generated POWER BOX WITH BOX OPERATIONS 7uncut_v3 (Autodesk Fusion 360 design; units mm, degrees)
Autodesk Fusion 360 part; units mm, degrees
(part 1 of 2)
sketch "b  stock" plane through (0, 0, 0) normal (0, 0, 1) x (1, 0, 0)
  line L0 (0, 0) -> (304.8, 0)
  line L1 (304.8, 0) -> (304.8, 609.6)
  line L2 (304.8, 609.6) -> (0, 609.6)
  line L3 (0, 609.6) -> (0, 0)
extrude "b  stock body extrude Feature" add sketch "b  stock" along normal blind 3.175 makes body 1
sketch "b  layout" plane through (0, 0, 0) normal (0, 0, 1) x (1, 0, 0)
  line L0 (0, 0) -> (90, 0)
  line L1 (90, 0) -> (90, 85)
  line L2 (90, 85) -> (0, 85)
  line L3 (0, 85) -> (0, 0)
  line L4 (92.01, 0) -> (182.01, 0)
  line L5 (182.01, 0) -> (182.01, 85)
  line L6 (182.01, 85) -> (92.01, 85)
  line L7 (92.01, 85) -> (92.01, 0)
  line L8 (184.02, 0) -> (234.02, 0)
  line L9 (234.02, 0) -> (234.02, 85)
  line L10 (234.02, 85) -> (184.02, 85)
  line L11 (184.02, 85) -> (184.02, 0)
  line L12 (236.03, 0) -> (286.03, 0)
  line L13 (286.03, 0) -> (286.03, 85)
  line L14 (286.03, 85) -> (236.03, 85)
  line L15 (236.03, 85) -> (236.03, 0)
  line L16 (0, 87.01) -> (90, 87.01)
  line L17 (90, 87.01) -> (90, 137.01)
  line L18 (90, 137.01) -> (0, 137.01)
  line L19 (0, 137.01) -> (0, 87.01)
  line L20 (92.01, 87.01) -> (182.01, 87.01)
  line L21 (182.01, 87.01) -> (182.01, 137.01)
  line L22 (182.01, 137.01) -> (92.01, 137.01)
  line L23 (92.01, 137.01) -> (92.01, 87.01)
sketch "top content" plane through (0, 0, 0) normal (0, 0, 1) x (1, 0, 0) in component "b top component"
  line L0 (0, 85) -> (90, 85) construction
  line L1 (90, 0) -> (0, 0) construction
  line L2 (14.1663, 44.1604) -> (78.1663, 44.1604) construction
  line L3 (78.1663, 44.1604) -> (78.1663, 63.1604) construction
  line L4 (78.1663, 63.1604) -> (14.1663, 63.1604) construction
  line L5 (14.1663, 63.1604) -> (14.1663, 44.1604) construction
  line L6 (0, 0) -> (0, 85) construction
  dimension "d1818" = 15
  dimension "d1163" = 90
  dimension "d1817" = 85
  constraint horizontal L0
  constraint perpendicular L1 L6
  measures "d1163" distance of L0.start L0.end
  measures "d1817" distance of L1.start L0.end
sketch "b top lines" plane through (0, 0, 0) normal (0, 0, 1) x (1, 0, 0) in component "b top component"
  line L0 (0, 0) -> (10.1, 0)
  line L1 (10.1, 0) -> (10.1, 3.175)
  line L2 (10.1, 3.175) -> (19.9, 3.175)
  line L3 (19.9, 3.175) -> (19.9, 0)
  line L4 (19.9, 0) -> (30.1, 0)
  line L5 (30.1, 0) -> (30.1, 3.175)
  line L6 (30.1, 3.175) -> (39.9, 3.175)
  line L7 (39.9, 3.175) -> (39.9, 0)
  line L8 (39.9, 0) -> (50.1, 0)
  line L9 (50.1, 0) -> (50.1, 3.175)
  line L10 (50.1, 3.175) -> (59.9, 3.175)
  line L11 (59.9, 3.175) -> (59.9, 0)
  line L12 (59.9, 0) -> (70.1, 0)
  line L13 (70.1, 0) -> (70.1, 3.175)
  line L14 (70.1, 3.175) -> (79.9, 3.175)
  line L15 (79.9, 3.175) -> (79.9, 0)
  line L16 (79.9, 0) -> (90, 0)
  line L17 (90, 0) -> (90, 17.6)
  line L18 (90, 17.6) -> (86.825, 17.6)
  line L19 (86.825, 17.6) -> (86.825, 27.4)
  line L20 (86.825, 27.4) -> (90, 27.4)
  line L21 (90, 27.4) -> (90, 37.6)
  line L22 (90, 37.6) -> (86.825, 37.6)
  line L23 (86.825, 37.6) -> (86.825, 47.4)
  line L24 (86.825, 47.4) -> (90, 47.4)
  line L25 (90, 47.4) -> (90, 57.6)
  line L26 (90, 57.6) -> (86.825, 57.6)
  line L27 (86.825, 57.6) -> (86.825, 67.4)
  line L28 (86.825, 67.4) -> (90, 67.4)
  line L29 (90, 67.4) -> (90, 85)
  line L30 (0, 85) -> (10.1, 85)
  line L31 (10.1, 85) -> (10.1, 81.825)
  line L32 (10.1, 81.825) -> (19.9, 81.825)
  line L33 (19.9, 81.825) -> (19.9, 85)
  line L34 (19.9, 85) -> (30.1, 85)
  line L35 (30.1, 85) -> (30.1, 81.825)
  line L36 (30.1, 81.825) -> (39.9, 81.825)
  line L37 (39.9, 81.825) -> (39.9, 85)
  line L38 (39.9, 85) -> (50.1, 85)
  line L39 (50.1, 85) -> (50.1, 81.825)
  line L40 (50.1, 81.825) -> (59.9, 81.825)
  line L41 (59.9, 81.825) -> (59.9, 85)
  line L42 (59.9, 85) -> (70.1, 85)
  line L43 (70.1, 85) -> (70.1, 81.825)
  line L44 (70.1, 81.825) -> (79.9, 81.825)
  line L45 (79.9, 81.825) -> (79.9, 85)
  line L46 (79.9, 85) -> (90, 85)
  line L47 (0, 0) -> (0, 17.6)
  line L48 (0, 17.6) -> (3.175, 17.6)
  line L49 (3.175, 17.6) -> (3.175, 27.4)
  line L50 (3.175, 27.4) -> (0, 27.4)
  line L51 (0, 27.4) -> (0, 37.6)
  line L52 (0, 37.6) -> (3.175, 37.6)
  line L53 (3.175, 37.6) -> (3.175, 47.4)
  line L54 (3.175, 47.4) -> (0, 47.4)
  line L55 (0, 47.4) -> (0, 57.6)
  line L56 (0, 57.6) -> (3.175, 57.6)
  line L57 (3.175, 57.6) -> (3.175, 67.4)
  line L58 (3.175, 67.4) -> (0, 67.4)
  line L59 (0, 67.4) -> (0, 85)
sketch "b top circles" plane through (0, 0, 0) normal (0, 0, 1) x (1, 0, 0) in component "b top component"
  circle A0 centre (10.6906, 2.4644) radius 1.005
  circle A1 centre (19.3094, 2.4644) radius 1.005
  circle A2 centre (30.6906, 2.4644) radius 1.005
  circle A3 centre (39.3094, 2.4644) radius 1.005
  circle A4 centre (50.6906, 2.4644) radius 1.005
  circle A5 centre (59.3094, 2.4644) radius 1.005
  circle A6 centre (70.6906, 2.4644) radius 1.005
  circle A7 centre (79.3094, 2.4644) radius 1.005
  circle A8 centre (87.5356, 18.1906) radius 1.005
  circle A9 centre (87.5356, 26.8094) radius 1.005
  circle A10 centre (87.5356, 38.1906) radius 1.005
  circle A11 centre (87.5356, 46.8094) radius 1.005
  circle A12 centre (87.5356, 58.1906) radius 1.005
  circle A13 centre (87.5356, 66.8094) radius 1.005
  circle A14 centre (10.6906, 82.5356) radius 1.005
  circle A15 centre (19.3094, 82.5356) radius 1.005
  circle A16 centre (30.6906, 82.5356) radius 1.005
  circle A17 centre (39.3094, 82.5356) radius 1.005
  circle A18 centre (50.6906, 82.5356) radius 1.005
  circle A19 centre (59.3094, 82.5356) radius 1.005
  circle A20 centre (70.6906, 82.5356) radius 1.005
  circle A21 centre (79.3094, 82.5356) radius 1.005
  circle A22 centre (2.4644, 18.1906) radius 1.005
  circle A23 centre (2.4644, 26.8094) radius 1.005
  circle A24 centre (2.4644, 38.1906) radius 1.005
  circle A25 centre (2.4644, 46.8094) radius 1.005
  circle A26 centre (2.4644, 58.1906) radius 1.005
  circle A27 centre (2.4644, 66.8094) radius 1.005
extrude "b top lines lines extrude Feature" add sketch "b top lines" along normal blind 3.175 separate body makes body 2 in component "b top component"
extrude "b top circles circles extrude Feature" add sketch "b top circles" along normal blind 3.175 separate body makes body 3 at (3.4644, 58.0906, 2.1167) makes body 4 at (3.4644, 38.0906, 2.1167) makes body 5 at (3.4644, 18.0906, 2.1167) makes body 6 at (69.7463, 82.8794, 2.1167) makes body 7 at (49.7463, 82.8794, 2.1167) makes body 8 at (31.6167, 82.926, 2.1167) makes body 9 at (9.7463, 82.8794, 2.1167) makes body 10 at (86.5913, 67.1531, 2.1167) makes body 11 at (87.2156, 45.8567, 1.0583) makes body 12 at (87.2156, 25.8567, 1.0583) makes body 13 at (78.9893, 1.5117, 1.0583) makes body 14 at (59.2843, 3.469, 2.1167) makes body 15 at (39.2843, 3.469, 2.1167) makes body 16 at (20.3094, 2.3643, 2.1167) makes body 17 at (31.6906, 2.3643, 2.1167) makes body 18 at (50.6656, 3.469, 2.1167) makes body 19 at (70.3706, 1.5117, 1.0583) makes body 20 at (87.2156, 17.238, 1.0583) makes body 21 at (87.2156, 37.238, 1.0583) makes body 22 at (87.2156, 57.238, 1.0583) makes body 23 at (11.6906, 2.3643, 2.1167) makes body 24 at (20.2354, 82.926, 2.1167) makes body 25 at (38.365, 82.8794, 2.1167) makes body 26 at (58.365, 82.8794, 2.1167) makes body 27 at (78.365, 82.8794, 2.1167) makes body 28 at (3.4644, 26.7093, 2.1167) makes body 29 at (3.4644, 46.7093, 2.1167) makes body 30 at (3.3904, 67.1997, 2.1167) in component "b top component"
combine "b top lines final combine feature" operation cut target body 2 tool bodies 3 4 5 6 7 8 9 10 11 12 13 14 15 16 17 18 19 20 21 22 23 24 25 26 27 28 29 30 in component "b top component"
sketch "bottom content" plane through (0, 0, 0) normal (0, 0, 1) x (1, 0, 0) in component "b bottom component"
  line L0 (92.01, 0) -> (182.01, 0) construction
  line L1 (182.01, 0) -> (182.01, 85) construction
  line L2 (182.01, 85) -> (92.01, 85) construction
  line L3 (92.01, 85) -> (92.01, 0) construction
  line L4 (182.01, 85) -> (182.01, 0) construction
  line L5 (182.01, 0) -> (92.01, 0) construction
  line L6 (92.01, 85) -> (182.01, 85) construction
  line L7 (92.01, 0) -> (92.01, 85) construction
  circle A0 centre (108.01, 55.5) radius 1.005
  circle A1 centre (172.01, 75) radius 1.005
  circle A2 centre (166.01, 55.5) radius 1.005
  circle A3 centre (166.01, 29.5) radius 1.005
  circle A4 centre (172.01, 10) radius 1.005
  circle A5 centre (102.01, 10) radius 1.005
  circle A6 centre (108.01, 29.5) radius 1.005
  circle A7 centre (102.01, 75) radius 1.005
  circle A8 centre (172.01, 75) radius 1.005
  point P0 (102.01, 75)
  point P1 (108.01, 55.5)
  point P2 (172.01, 75)
  point P3 (166.01, 29.5)
  point P4 (166.01, 55.5)
  point P5 (172.01, 10)
  point P6 (102.01, 10)
  point P7 (108.01, 29.5)
  point P8 (182.01, 85)
  dimension "d467" = 90
  dimension "d468" = 85
  dimension "d469" = 10
  dimension "d470" = 10
  dimension "d471" = 29.5
  dimension "d472" = 16
  dimension "d473" = 2.01
  dimension "d474" = 2.01
  constraint horizontal L5
  constraint perpendicular L5 L7
  constraint parallel L5 L6
  constraint coincident L1.end L2.start
  constraint vertical L4
  constraint coincident P1 A0.centre
  constraint coincident P2 A1.centre
  constraint coincident P4 A2.centre
  constraint coincident P3 A3.centre
  constraint coincident P5 A4.centre
  constraint coincident P6 A5.centre
  constraint coincident P7 A6.centre
  constraint coincident P0 A7.centre
  constraint concentric A1 A8
  constraint equal A0 A2
  constraint equal A7 A8
  constraint equal A0 A6
  constraint equal A0 A3
  constraint equal A3 A5
  constraint equal A3 A8
  constraint equal A2 A4
  measures "d467" distance of L1.end L2.end
  measures "d468" distance of L0.start L2.end
  measures "d469" distance of P0 L6
  measures "d470" distance of P0 L7
  measures "d471" distance of P1 L6
  measures "d472" distance of P7 L7
  measures "d473" diameter of A0
  measures "d474" diameter of A1
sketch "b bottom lines" plane through (0, 0, 0) normal (0, 0, 1) x (1, 0, 0) in component "b bottom component"
  line L0 (92.01, 0) -> (102.11, 0)
  line L1 (102.11, 0) -> (102.11, 3.175)
  line L2 (102.11, 3.175) -> (111.91, 3.175)
  line L3 (111.91, 3.175) -> (111.91, 0)
  line L4 (111.91, 0) -> (122.11, 0)
  line L5 (122.11, 0) -> (122.11, 3.175)
  line L6 (122.11, 3.175) -> (131.91, 3.175)
  line L7 (131.91, 3.175) -> (131.91, 0)
  line L8 (131.91, 0) -> (142.11, 0)
  line L9 (142.11, 0) -> (142.11, 3.175)
  line L10 (142.11, 3.175) -> (151.91, 3.175)
  line L11 (151.91, 3.175) -> (151.91, 0)
  line L12 (151.91, 0) -> (162.11, 0)
  line L13 (162.11, 0) -> (162.11, 3.175)
  line L14 (162.11, 3.175) -> (171.91, 3.175)
  line L15 (171.91, 3.175) -> (171.91, 0)
  line L16 (171.91, 0) -> (182.01, 0)
  line L17 (182.01, 0) -> (182.01, 17.6)
  line L18 (182.01, 17.6) -> (178.835, 17.6)
  line L19 (178.835, 17.6) -> (178.835, 27.4)
  line L20 (178.835, 27.4) -> (182.01, 27.4)
  line L21 (182.01, 27.4) -> (182.01, 37.6)
  line L22 (182.01, 37.6) -> (178.835, 37.6)
  line L23 (178.835, 37.6) -> (178.835, 47.4)
  line L24 (178.835, 47.4) -> (182.01, 47.4)
  line L25 (182.01, 47.4) -> (182.01, 57.6)
  line L26 (182.01, 57.6) -> (178.835, 57.6)
  line L27 (178.835, 57.6) -> (178.835, 67.4)
  line L28 (178.835, 67.4) -> (182.01, 67.4)
  line L29 (182.01, 67.4) -> (182.01, 85)
  line L30 (92.01, 85) -> (102.11, 85)
  line L31 (102.11, 85) -> (102.11, 81.825)
  line L32 (102.11, 81.825) -> (111.91, 81.825)
  line L33 (111.91, 81.825) -> (111.91, 85)
  line L34 (111.91, 85) -> (122.11, 85)
  line L35 (122.11, 85) -> (122.11, 81.825)
  line L36 (122.11, 81.825) -> (131.91, 81.825)
  line L37 (131.91, 81.825) -> (131.91, 85)
  line L38 (131.91, 85) -> (142.11, 85)
  line L39 (142.11, 85) -> (142.11, 81.825)
  line L40 (142.11, 81.825) -> (151.91, 81.825)
  line L41 (151.91, 81.825) -> (151.91, 85)
  line L42 (151.91, 85) -> (162.11, 85)
  line L43 (162.11, 85) -> (162.11, 81.825)
  line L44 (162.11, 81.825) -> (171.91, 81.825)
  line L45 (171.91, 81.825) -> (171.91, 85)
  line L46 (171.91, 85) -> (182.01, 85)
  line L47 (92.01, 0) -> (92.01, 17.6)
  line L48 (92.01, 17.6) -> (95.185, 17.6)
  line L49 (95.185, 17.6) -> (95.185, 27.4)
  line L50 (95.185, 27.4) -> (92.01, 27.4)
  line L51 (92.01, 27.4) -> (92.01, 37.6)
  line L52 (92.01, 37.6) -> (95.185, 37.6)
  line L53 (95.185, 37.6) -> (95.185, 47.4)
  line L54 (95.185, 47.4) -> (92.01, 47.4)
  line L55 (92.01, 47.4) -> (92.01, 57.6)
  line L56 (92.01, 57.6) -> (95.185, 57.6)
  line L57 (95.185, 57.6) -> (95.185, 67.4)
  line L58 (95.185, 67.4) -> (92.01, 67.4)
  line L59 (92.01, 67.4) -> (92.01, 85)
sketch "b bottom circles" plane through (0, 0, 0) normal (0, 0, 1) x (1, 0, 0) in component "b bottom component"
  circle A0 centre (102.7006, 2.4644) radius 1.005
  circle A1 centre (111.3194, 2.4644) radius 1.005
  circle A2 centre (122.7006, 2.4644) radius 1.005
  circle A3 centre (131.3194, 2.4644) radius 1.005
  circle A4 centre (142.7006, 2.4644) radius 1.005
  circle A5 centre (151.3194, 2.4644) radius 1.005
  circle A6 centre (162.7006, 2.4644) radius 1.005
  circle A7 centre (171.3194, 2.4644) radius 1.005
  circle A8 centre (179.5456, 18.1906) radius 1.005
  circle A9 centre (179.5456, 26.8094) radius 1.005
  circle A10 centre (179.5456, 38.1906) radius 1.005
  circle A11 centre (179.5456, 46.8094) radius 1.005
  circle A12 centre (179.5456, 58.1906) radius 1.005
  circle A13 centre (179.5456, 66.8094) radius 1.005
  circle A14 centre (102.7006, 82.5356) radius 1.005
  circle A15 centre (111.3194, 82.5356) radius 1.005
  circle A16 centre (122.7006, 82.5356) radius 1.005
  circle A17 centre (131.3194, 82.5356) radius 1.005
  circle A18 centre (142.7006, 82.5356) radius 1.005
  circle A19 centre (151.3194, 82.5356) radius 1.005
  circle A20 centre (162.7006, 82.5356) radius 1.005
  circle A21 centre (171.3194, 82.5356) radius 1.005
  circle A22 centre (94.4744, 18.1906) radius 1.005
  circle A23 centre (94.4744, 26.8094) radius 1.005
  circle A24 centre (94.4744, 38.1906) radius 1.005
  circle A25 centre (94.4744, 46.8094) radius 1.005
  circle A26 centre (94.4744, 58.1906) radius 1.005
  circle A27 centre (94.4744, 66.8094) radius 1.005
extrude "b bottom lines lines extrude Feature" add sketch "b bottom lines" along normal blind 3.175 separate body makes body 31 in component "b bottom component"
extrude "b bottom circles circles extrude Feature" add sketch "b bottom circles" along normal blind 3.175 separate body makes body 32 at (94.1543, 57.238, 1.0583) makes body 33 at (94.1543, 37.238, 1.0583) makes body 34 at (94.1543, 17.238, 1.0583) makes body 35 at (161.7563, 82.8794, 2.1167) makes body 36 at (141.7563, 82.8794, 2.1167) makes body 37 at (121.7563, 82.8794, 2.1167) makes body 38 at (101.7563, 82.8794, 2.1167) makes body 39 at (178.6013, 67.1531, 2.1167) makes body 40 at (180.4717, 47.1997, 2.1167) makes body 41 at (179.959, 27.7254, 2.1167) makes body 42 at (170.906, 3.3804, 2.1167) makes body 43 at (150.906, 3.3804, 2.1167) makes body 44 at (130.906, 3.3804, 2.1167) makes body 45 at (110.9993, 1.5117, 1.0583) makes body 46 at (122.3806, 1.5117, 1.0583) makes body 47 at (142.2873, 3.3804, 2.1167) makes body 48 at (162.2873, 3.3804, 2.1167) makes body 49 at (179.959, 19.1067, 2.1167) makes body 50 at (180.4717, 38.581, 2.1167) makes body 51 at (180.4717, 58.581, 2.1167) makes body 52 at (102.3806, 1.5117, 1.0583) makes body 53 at (110.375, 82.8794, 2.1167) makes body 54 at (130.375, 82.8794, 2.1167) makes body 55 at (150.375, 82.8794, 2.1167) makes body 56 at (170.375, 82.8794, 2.1167) makes body 57 at (94.1543, 25.8567, 1.0583) makes body 58 at (94.1543, 45.8567, 1.0583) makes body 59 at (93.53, 67.1531, 2.1167) in component "b bottom component"
combine "b bottom lines final combine feature" operation cut target body 31 tool bodies 32 33 34 35 36 37 38 39 40 41 42 43 44 45 46 47 48 49 50 51 52 53 54 55 56 57 58 59 in component "b bottom component"
sketch "left content" plane through (0, 0, 0) normal (0, 0, 1) x (1, 0, 0) in component "b left component"
  line L0 (184.02, 0) -> (234.02, 0) construction
  line L1 (234.02, 0) -> (234.02, 85) construction
  line L2 (234.02, 85) -> (184.02, 85) construction
  line L3 (184.02, 85) -> (184.02, 0) construction
  circle A0 centre (205.99, 40) radius 1.5
  circle A1 centre (205.99, 52) radius 1.5
  circle A2 centre (193.99, 52) radius 1.5
  circle A3 centre (193.99, 64) radius 1.5
  circle A4 centre (205.99, 64) radius 0
  circle A5 centre (199.99, 16) radius 1.5
  circle A6 centre (199.99, 52) radius 1.5
  circle A7 centre (199.99, 64) radius 0
  circle A8 centre (199.99, 46) radius 1.5
  circle A9 centre (193.99, 28) radius 1.5
  circle A10 centre (199.99, 22) radius 1.5
  circle A11 centre (205.99, 28) radius 1.5
  circle A12 centre (199.99, 28) radius 1.5
  circle A13 centre (193.99, 58) radius 1.5
  circle A14 centre (205.99, 22) radius 1.5
  circle A15 centre (205.99, 10) radius 1.5
  circle A16 centre (193.99, 22) radius 1.5
  circle A17 centre (205.99, 34) radius 1.5
  circle A18 centre (193.99, 34) radius 1.5
  circle A19 centre (199.99, 58) radius 1.5
  circle A20 centre (193.99, 16) radius 1.5
  circle A21 centre (199.99, 10) radius 1.5
  circle A22 centre (193.99, 64) radius 0
  circle A23 centre (199.99, 34) radius 1.5
  circle A24 centre (199.99, 64) radius 1.5
  circle A25 centre (205.99, 46) radius 1.5
  circle A26 centre (193.99, 10) radius 1.5
  circle A27 centre (193.99, 46) radius 1.5
  circle A28 centre (193.99, 40) radius 1.5
  circle A29 centre (205.99, 58) radius 1.5
  circle A30 centre (205.99, 16) radius 1.5
  circle A31 centre (199.99, 40) radius 1.5
  circle A32 centre (205.99, 64) radius 1.5
  line L4 (184.02, 0) -> (234.02, 0)
  point P0 (193.99, 70)
  point P1 (199.99, 70)
  point P2 (211.99, 46)
  point P3 (211.99, 52)
  point P4 (211.99, 64)
  point P5 (205.99, 70)
  point P6 (211.99, 58)
  point P7 (211.99, 70)
  point P8 (194.02, 10)
  dimension "d487" = 6
  dimension "d488" = 6
  dimension "d489" = 10
  dimension "d490" = 10
  measures "d489" distance of L3 P8
  measures "d490" distance of A26.centre L4
sketch "b left lines" plane through (0, 0, 0) normal (0, 0, 1) x (1, 0, 0) in component "b left component"
  line L0 (187.195, 0) -> (194.12, 0)
  line L1 (194.12, 0) -> (194.12, 3.175)
  line L2 (194.12, 3.175) -> (203.92, 3.175)
  line L3 (203.92, 3.175) -> (203.92, 0)
  line L4 (203.92, 0) -> (214.12, 0)
  line L5 (214.12, 0) -> (214.12, 3.175)
  line L6 (214.12, 3.175) -> (223.92, 3.175)
  line L7 (223.92, 3.175) -> (223.92, 0)
  line L8 (223.92, 0) -> (230.845, 0)
  line L9 (230.845, 0) -> (230.845, 17.4)
  line L10 (230.845, 17.4) -> (234.02, 17.4)
  line L11 (234.02, 17.4) -> (234.02, 27.6)
  line L12 (234.02, 27.6) -> (230.845, 27.6)
  line L13 (230.845, 27.6) -> (230.845, 37.4)
  line L14 (230.845, 37.4) -> (234.02, 37.4)
  line L15 (234.02, 37.4) -> (234.02, 47.6)
  line L16 (234.02, 47.6) -> (230.845, 47.6)
  line L17 (230.845, 47.6) -> (230.845, 57.4)
  line L18 (230.845, 57.4) -> (234.02, 57.4)
  line L19 (234.02, 57.4) -> (234.02, 67.6)
  line L20 (234.02, 67.6) -> (230.845, 67.6)
  line L21 (230.845, 67.6) -> (230.845, 85)
  line L22 (187.195, 85) -> (194.12, 85)
  line L23 (194.12, 85) -> (194.12, 81.825)
  line L24 (194.12, 81.825) -> (203.92, 81.825)
  line L25 (203.92, 81.825) -> (203.92, 85)
  line L26 (203.92, 85) -> (214.12, 85)
  line L27 (214.12, 85) -> (214.12, 81.825)
  line L28 (214.12, 81.825) -> (223.92, 81.825)
  line L29 (223.92, 81.825) -> (223.92, 85)
  line L30 (223.92, 85) -> (230.845, 85)
  line L31 (187.195, 0) -> (187.195, 17.4)
  line L32 (187.195, 17.4) -> (184.02, 17.4)
  line L33 (184.02, 17.4) -> (184.02, 27.6)
  line L34 (184.02, 27.6) -> (187.195, 27.6)
  line L35 (187.195, 27.6) -> (187.195, 37.4)
  line L36 (187.195, 37.4) -> (184.02, 37.4)
  line L37 (184.02, 37.4) -> (184.02, 47.6)
  line L38 (184.02, 47.6) -> (187.195, 47.6)
  line L39 (187.195, 47.6) -> (187.195, 57.4)
  line L40 (187.195, 57.4) -> (184.02, 57.4)
  line L41 (184.02, 57.4) -> (184.02, 67.6)
  line L42 (184.02, 67.6) -> (187.195, 67.6)
  line L43 (187.195, 67.6) -> (187.195, 85)
sketch "b left circles" plane through (0, 0, 0) normal (0, 0, 1) x (1, 0, 0) in component "b left component"
  circle A0 centre (194.7106, 2.4644) radius 1.005
  circle A1 centre (203.3294, 2.4644) radius 1.005
  circle A2 centre (214.7106, 2.4644) radius 1.005
  circle A3 centre (223.3294, 2.4644) radius 1.005
  circle A4 centre (231.5556, 16.8094) radius 1.005
  circle A5 centre (231.5556, 28.1906) radius 1.005
  circle A6 centre (231.5556, 36.8094) radius 1.005
  circle A7 centre (231.5556, 48.1906) radius 1.005
  circle A8 centre (231.5556, 56.8094) radius 1.005
  circle A9 centre (231.5556, 68.1906) radius 1.005
  circle A10 centre (194.7106, 82.5356) radius 1.005
  circle A11 centre (203.3294, 82.5356) radius 1.005
  circle A12 centre (214.7106, 82.5356) radius 1.005
  circle A13 centre (223.3294, 82.5356) radius 1.005
  circle A14 centre (186.4844, 16.8094) radius 1.005
  circle A15 centre (186.4844, 28.1906) radius 1.005
  circle A16 centre (186.4844, 36.8094) radius 1.005
  circle A17 centre (186.4844, 48.1906) radius 1.005
  circle A18 centre (186.4844, 56.8094) radius 1.005
  circle A19 centre (186.4844, 68.1906) radius 1.005
extrude "b left lines lines extrude Feature" add sketch "b left lines" along normal blind 3.175 separate body makes body 60 in component "b left component"
extrude "b left circles circles extrude Feature" add sketch "b left circles" along normal blind 3.175 separate body makes body 61 at (187.4104, 57.1997, 2.1167) makes body 62 at (187.4104, 37.1997, 2.1167) makes body 63 at (186.8977, 17.7254, 2.1167) makes body 64 at (213.7663, 82.8794, 2.1167) makes body 65 at (193.7663, 82.8794, 2.1167) makes body 66 at (230.6113, 68.5344, 2.1167) makes body 67 at (232.4817, 48.581, 2.1167) makes body 68 at (231.969, 29.1067, 2.1167) makes body 69 at (222.916, 3.3804, 2.1167) makes body 70 at (202.916, 3.3804, 2.1167) makes body 71 at (214.2973, 3.3804, 2.1167) makes body 72 at (231.969, 17.7254, 2.1167) makes body 73 at (232.4817, 37.1997, 2.1167) makes body 74 at (232.4817, 57.1997, 2.1167) makes body 75 at (194.2973, 3.3804, 2.1167) makes body 76 at (202.385, 82.8794, 2.1167) makes body 77 at (222.385, 82.8794, 2.1167) makes body 78 at (186.8977, 29.1067, 2.1167) makes body 79 at (187.4104, 48.581, 2.1167) makes body 80 at (185.54, 68.5344, 2.1167) in component "b left component"
combine "b left lines final combine feature" operation cut target body 60 tool bodies 61 62 63 64 65 66 67 68 69 70 71 72 73 74 75 76 77 78 79 80 in component "b left component"
sketch "right content" plane through (0, 0, 0) normal (0, 0, 1) x (1, 0, 0) in component "b right component"
  line L0 (236.03, 0) -> (286.03, 0) construction
  line L1 (286.03, 0) -> (286.03, 85) construction
  line L2 (286.03, 85) -> (236.03, 85) construction
  circle A0 centre (257.99, 64) radius 0
  circle A1 centre (251.99, 64) radius 0
  circle A2 centre (245.99, 64) radius 0
  circle A3 centre (246.03, 10) radius 0
  circle A4 centre (245.99, 10) radius 1.5
  circle A5 centre (263.99, 46) radius 0
  circle A6 centre (263.99, 52) radius 0
  circle A7 centre (263.99, 58) radius 0
  circle A8 centre (263.99, 64) radius 0
  circle A9 centre (245.99, 70) radius 0
  circle A10 centre (251.99, 70) radius 0
  circle A11 centre (257.99, 70) radius 0
  circle A12 centre (263.99, 70) radius 0
  circle A13 centre (251.99, 10) radius 1.5
  circle A14 centre (257.99, 10) radius 1.5
  circle A15 centre (245.99, 16) radius 1.5
  circle A16 centre (251.99, 16) radius 1.5
  circle A17 centre (257.99, 16) radius 1.5
  circle A18 centre (245.99, 22) radius 1.5
  circle A19 centre (251.99, 22) radius 1.5
  circle A20 centre (257.99, 22) radius 1.5
  circle A21 centre (245.99, 28) radius 1.5
  circle A22 centre (251.99, 28) radius 1.5
  circle A23 centre (257.99, 28) radius 1.5
  circle A24 centre (245.99, 34) radius 1.5
  circle A25 centre (251.99, 34) radius 1.5
  circle A26 centre (257.99, 34) radius 1.5
  circle A27 centre (245.99, 40) radius 1.5
  circle A28 centre (251.99, 40) radius 1.5
  circle A29 centre (257.99, 40) radius 1.5
  circle A30 centre (245.99, 46) radius 1.5
  circle A31 centre (251.99, 46) radius 1.5
  circle A32 centre (257.99, 46) radius 1.5
  circle A33 centre (245.99, 52) radius 1.5
  circle A34 centre (251.99, 52) radius 1.5
  circle A35 centre (257.99, 52) radius 1.5
  circle A36 centre (245.99, 58) radius 1.5
  circle A37 centre (251.99, 58) radius 1.5
  circle A38 centre (257.99, 58) radius 1.5
  circle A39 centre (245.99, 64) radius 1.5
  circle A40 centre (251.99, 64) radius 1.5
  circle A41 centre (257.99, 64) radius 1.5
  line L3 (236.03, 85) -> (236.03, 0)
  point P0 (-142.01, 0)
  point P1 (-117.01, 0)
  dimension "d479" = 0
  dimension "d483" = 6
  dimension "d484" = 6
  dimension "d491" = 10
  dimension "d494" = 10
  measures "d479" diameter of A3
  measures "d491" vertical distance of L0.start A3.centre
  measures "d494" distance of A3.centre L3
sketch "b right lines" plane through (0, 0, 0) normal (0, 0, 1) x (1, 0, 0) in component "b right component"
  line L0 (239.205, 0) -> (246.13, 0)
  line L1 (246.13, 0) -> (246.13, 3.175)
  line L2 (246.13, 3.175) -> (255.93, 3.175)
  line L3 (255.93, 3.175) -> (255.93, 0)
  line L4 (255.93, 0) -> (266.13, 0)
  line L5 (266.13, 0) -> (266.13, 3.175)
  line L6 (266.13, 3.175) -> (275.93, 3.175)
  line L7 (275.93, 3.175) -> (275.93, 0)
  line L8 (275.93, 0) -> (282.855, 0)
  line L9 (282.855, 0) -> (282.855, 17.4)
  line L10 (282.855, 17.4) -> (286.03, 17.4)
  line L11 (286.03, 17.4) -> (286.03, 27.6)
  line L12 (286.03, 27.6) -> (282.855, 27.6)
  line L13 (282.855, 27.6) -> (282.855, 37.4)
  line L14 (282.855, 37.4) -> (286.03, 37.4)
  line L15 (286.03, 37.4) -> (286.03, 47.6)
  line L16 (286.03, 47.6) -> (282.855, 47.6)
  line L17 (282.855, 47.6) -> (282.855, 57.4)
  line L18 (282.855, 57.4) -> (286.03, 57.4)
  line L19 (286.03, 57.4) -> (286.03, 67.6)
  line L20 (286.03, 67.6) -> (282.855, 67.6)
  line L21 (282.855, 67.6) -> (282.855, 85)
  line L22 (239.205, 85) -> (246.13, 85)
  line L23 (246.13, 85) -> (246.13, 81.825)
  line L24 (246.13, 81.825) -> (255.93, 81.825)
  line L25 (255.93, 81.825) -> (255.93, 85)
  line L26 (255.93, 85) -> (266.13, 85)
  line L27 (266.13, 85) -> (266.13, 81.825)
  line L28 (266.13, 81.825) -> (275.93, 81.825)
  line L29 (275.93, 81.825) -> (275.93, 85)
  line L30 (275.93, 85) -> (282.855, 85)
  line L31 (239.205, 0) -> (239.205, 17.4)
  line L32 (239.205, 17.4) -> (236.03, 17.4)
  line L33 (236.03, 17.4) -> (236.03, 27.6)
  line L34 (236.03, 27.6) -> (239.205, 27.6)
  line L35 (239.205, 27.6) -> (239.205, 37.4)
  line L36 (239.205, 37.4) -> (236.03, 37.4)
  line L37 (236.03, 37.4) -> (236.03, 47.6)
  line L38 (236.03, 47.6) -> (239.205, 47.6)
  line L39 (239.205, 47.6) -> (239.205, 57.4)
  line L40 (239.205, 57.4) -> (236.03, 57.4)
  line L41 (236.03, 57.4) -> (236.03, 67.6)
  line L42 (236.03, 67.6) -> (239.205, 67.6)
  line L43 (239.205, 67.6) -> (239.205, 85)
sketch "b right circles" plane through (0, 0, 0) normal (0, 0, 1) x (1, 0, 0) in component "b right component"
  circle A0 centre (246.7206, 2.4644) radius 1.005
  circle A1 centre (255.3394, 2.4644) radius 1.005
  circle A2 centre (266.7206, 2.4644) radius 1.005
  circle A3 centre (275.3394, 2.4644) radius 1.005
  circle A4 centre (283.5656, 16.8094) radius 1.005
  circle A5 centre (283.5656, 28.1906) radius 1.005
  circle A6 centre (283.5656, 36.8094) radius 1.005
  circle A7 centre (283.5656, 48.1906) radius 1.005
  circle A8 centre (283.5656, 56.8094) radius 1.005
  circle A9 centre (283.5656, 68.1906) radius 1.005
  circle A10 centre (246.7206, 82.5356) radius 1.005
  circle A11 centre (255.3394, 82.5356) radius 1.005
  circle A12 centre (266.7206, 82.5356) radius 1.005
  circle A13 centre (275.3394, 82.5356) radius 1.005
  circle A14 centre (238.4944, 16.8094) radius 1.005
  circle A15 centre (238.4944, 28.1906) radius 1.005
  circle A16 centre (238.4944, 36.8094) radius 1.005
  circle A17 centre (238.4944, 48.1906) radius 1.005
  circle A18 centre (238.4944, 56.8094) radius 1.005
  circle A19 centre (238.4944, 68.1906) radius 1.005
extrude "b right lines lines extrude Feature" add sketch "b right lines" along normal blind 3.175 separate body makes body 81 in component "b right component"
extrude "b right circles circles extrude Feature" add sketch "b right circles" along normal blind 3.175 separate body makes body 82 at (239.4204, 57.1997, 2.1167) makes body 83 at (239.4204, 37.1997, 2.1167) makes body 84 at (238.9077, 17.7254, 2.1167) makes body 85 at (266.9928, 83.5031, 2.1167) makes body 86 at (245.7763, 82.8794, 2.1167) makes body 87 at (283.8378, 69.1581, 2.1167) makes body 88 at (283.8378, 49.1581, 2.1167) makes body 89 at (283.8378, 29.1581, 2.1167) makes body 90 at (275.6116, 3.4318, 2.1167) makes body 91 at (256.1092, 3.1104, 2.1167) makes body 92 at (266.9928, 3.4318, 2.1167) makes body 93 at (283.8378, 17.7768, 2.1167) makes body 94 at (283.8378, 37.7768, 2.1167) makes body 95 at (283.8378, 57.7768, 2.1167) makes body 96 at (246.3073, 3.3804, 2.1167) makes body 97 at (254.395, 82.8794, 2.1167) makes body 98 at (275.6116, 83.5031, 2.1167) makes body 99 at (238.9077, 29.1067, 2.1167) makes body 100 at (239.4204, 48.581, 2.1167) makes body 101 at (237.55, 68.5344, 2.1167) in component "b right component"
combine "b right lines final combine feature" operation cut target body 81 tool bodies 82 83 84 85 86 87 88 89 90 91 92 93 94 95 96 97 98 99 100 101 in component "b right component"
sketch "front content" plane through (0, 0, 0) normal (0, 0, 1) x (1, 0, 0) in component "b front component"
  line L0 (53.5, 95.01) -> (53.5, 105.31)
  circle A0 centre (13, 101.01) radius 6
  circle A1 centre (37, 101.01) radius 6
  line L1 (76.2, 105.31) -> (76.2, 95.01)
  line L2 (26.5, 128.31) -> (26.5, 118.01)
  line L3 (26.5, 118.01) -> (12, 118.01)
  line L4 (90, 137.01) -> (0, 137.01) construction
  circle A2 centre (65, 122.51) radius 3.5
  line L5 (76.2, 95.01) -> (53.5, 95.01)
  line L6 (53.5, 105.31) -> (76.2, 105.31)
  line L7 (90, 87.01) -> (90, 137.01) construction
  line L8 (0, 87.01) -> (0, 137.01) construction
  line L9 (12, 128.31) -> (26.5, 128.31)
  line L10 (12, 118.01) -> (12, 128.31)
  line L11 (0, 87.01) -> (90, 87.01) construction
  dimension "d230" = 90
  dimension "d231" = 50
  dimension "d232" = 12
  dimension "d233" = 24
  dimension "d234" = 14
  dimension "d235" = 13
  dimension "d236" = 14.5
  dimension "d237" = 10.3
  dimension "d238" = 31
  dimension "d239" = 12
  dimension "d240" = 7
  dimension "d241" = 25
  dimension "d242" = 14.5
  dimension "d243" = 22.7
  dimension "d244" = 10.3
  dimension "d245" = 13.8
  dimension "d246" = 8
  constraint perpendicular L4 L8
  constraint equal A0 A1
  measures "d230" distance of L7.start L8.start
  measures "d231" distance of L8.start L4.end
  measures "d232" diameter of A1
  measures "d233" distance of A1.centre A0.centre
  measures "d234" distance of A1.centre L11
  measures "d235" distance of A0.centre L8
  measures "d236" distance of L2.end L3.end
  measures "d237" distance of L2.end L2.start
  measures "d238" distance of L3 L11
  measures "d239" distance of L8 L10
  measures "d240" diameter of A2
  measures "d241" distance of A2.centre L7
  measures "d242" distance of A2.centre L4
  measures "d243" distance of L1.end L0.start
  measures "d244" distance of L1.start L1.end
  measures "d245" distance of L1 L7
  measures "d246" distance of L5 L11
sketch "b front lines" plane through (0, 0, 0) normal (0, 0, 1) x (1, 0, 0) in component "b front component"
  line L0 (3.175, 90.185) -> (9.9, 90.185)
  line L1 (9.9, 90.185) -> (9.9, 87.01)
  line L2 (9.9, 87.01) -> (20.1, 87.01)
  line L3 (20.1, 87.01) -> (20.1, 90.185)
  line L4 (20.1, 90.185) -> (29.9, 90.185)
  line L5 (29.9, 90.185) -> (29.9, 87.01)
  line L6 (29.9, 87.01) -> (40.1, 87.01)
  line L7 (40.1, 87.01) -> (40.1, 90.185)
  line L8 (40.1, 90.185) -> (49.9, 90.185)
  line L9 (49.9, 90.185) -> (49.9, 87.01)
  line L10 (49.9, 87.01) -> (60.1, 87.01)
  line L11 (60.1, 87.01) -> (60.1, 90.185)
  line L12 (60.1, 90.185) -> (69.9, 90.185)
  line L13 (69.9, 90.185) -> (69.9, 87.01)
  line L14 (69.9, 87.01) -> (80.1, 87.01)
  line L15 (80.1, 87.01) -> (80.1, 90.185)
  line L16 (80.1, 90.185) -> (86.825, 90.185)
  line L17 (86.825, 90.185) -> (86.825, 96.91)
  line L18 (86.825, 96.91) -> (90, 96.91)
  line L19 (90, 96.91) -> (90, 107.11)
  line L20 (90, 107.11) -> (86.825, 107.11)
  line L21 (86.825, 107.11) -> (86.825, 116.91)
  line L22 (86.825, 116.91) -> (90, 116.91)
  line L23 (90, 116.91) -> (90, 127.11)
  line L24 (90, 127.11) -> (86.825, 127.11)
  line L25 (86.825, 127.11) -> (86.825, 133.835)
  line L26 (3.175, 133.835) -> (9.9, 133.835)
  line L27 (9.9, 133.835) -> (9.9, 137.01)
  line L28 (9.9, 137.01) -> (20.1, 137.01)
  line L29 (20.1, 137.01) -> (20.1, 133.835)
  line L30 (20.1, 133.835) -> (29.9, 133.835)
  line L31 (29.9, 133.835) -> (29.9, 137.01)
  line L32 (29.9, 137.01) -> (40.1, 137.01)
  line L33 (40.1, 137.01) -> (40.1, 133.835)
  line L34 (40.1, 133.835) -> (49.9, 133.835)
  line L35 (49.9, 133.835) -> (49.9, 137.01)
  line L36 (49.9, 137.01) -> (60.1, 137.01)
  line L37 (60.1, 137.01) -> (60.1, 133.835)
  line L38 (60.1, 133.835) -> (69.9, 133.835)
  line L39 (69.9, 133.835) -> (69.9, 137.01)
  line L40 (69.9, 137.01) -> (80.1, 137.01)
  line L41 (80.1, 137.01) -> (80.1, 133.835)
  line L42 (80.1, 133.835) -> (86.825, 133.835)
  line L43 (3.175, 90.185) -> (3.175, 96.91)
  line L44 (3.175, 96.91) -> (0, 96.91)
  line L45 (0, 96.91) -> (0, 107.11)
  line L46 (0, 107.11) -> (3.175, 107.11)
  line L47 (3.175, 107.11) -> (3.175, 116.91)
  line L48 (3.175, 116.91) -> (0, 116.91)
  line L49 (0, 116.91) -> (0, 127.11)
  line L50 (0, 127.11) -> (3.175, 127.11)
  line L51 (3.175, 127.11) -> (3.175, 133.835)
sketch "b front circles" plane through (0, 0, 0) normal (0, 0, 1) x (1, 0, 0) in component "b front component"
  circle A0 centre (9.3094, 89.4744) radius 1.005
  circle A1 centre (20.6906, 89.4744) radius 1.005
  circle A2 centre (29.3094, 89.4744) radius 1.005
  circle A3 centre (40.6906, 89.4744) radius 1.005
  circle A4 centre (49.3094, 89.4744) radius 1.005
  circle A5 centre (60.6906, 89.4744) radius 1.005
  circle A6 centre (69.3094, 89.4744) radius 1.005
  circle A7 centre (80.6906, 89.4744) radius 1.005
  circle A8 centre (87.5356, 96.3194) radius 1.005
  circle A9 centre (87.5356, 107.7006) radius 1.005
  circle A10 centre (87.5356, 116.3194) radius 1.005
  circle A11 centre (87.5356, 127.7006) radius 1.005
  circle A12 centre (9.3094, 134.5456) radius 1.005
  circle A13 centre (20.6906, 134.5456) radius 1.005
  circle A14 centre (29.3094, 134.5456) radius 1.005
  circle A15 centre (40.6906, 134.5456) radius 1.005
  circle A16 centre (49.3094, 134.5456) radius 1.005
  circle A17 centre (60.6906, 134.5456) radius 1.005
  circle A18 centre (69.3094, 134.5456) radius 1.005
  circle A19 centre (80.6906, 134.5456) radius 1.005
  circle A20 centre (2.4644, 96.3194) radius 1.005
  circle A21 centre (2.4644, 107.7006) radius 1.005
  circle A22 centre (2.4644, 116.3194) radius 1.005
  circle A23 centre (2.4644, 127.7006) radius 1.005
extrude "b front lines lines extrude Feature" add sketch "b front lines" along normal blind 3.175 separate body makes body 102 in component "b front component"
extrude "b front circles circles extrude Feature" add sketch "b front circles" along normal blind 3.175 separate body makes body 103 at (3.3904, 116.7097, 2.1167) makes body 104 at (3.3904, 96.7097, 2.1167) makes body 105 at (70.0792, 135.1916, 2.1167) makes body 106 at (50.0792, 135.1916, 2.1167) makes body 107 at (29.7227, 135.4617, 2.1167) makes body 108 at (9.7227, 135.4617, 2.1167) makes body 109 at (86.5913, 128.0444, 2.1167) makes body 110 at (86.5913, 108.0444, 2.1167) makes body 111 at (79.7463, 89.8181, 2.1167) makes body 112 at (59.7463, 89.8181, 2.1167) makes body 113 at (39.7463, 89.8181, 2.1167) makes body 114 at (21.6167, 89.8647, 2.1167) makes body 115 at (30.2354, 89.8647, 2.1167) makes body 116 at (48.365, 89.8181, 2.1167) makes body 117 at (68.365, 89.8181, 2.1167) makes body 118 at (86.5913, 96.6631, 2.1167) makes body 119 at (86.5913, 116.6631, 2.1167) makes body 120 at (8.365, 89.8181, 2.1167) makes body 121 at (19.9208, 133.8996, 2.1167) makes body 122 at (41.4605, 135.1916, 2.1167) makes body 123 at (61.4605, 135.1916, 2.1167) makes body 124 at (81.4605, 135.1916, 2.1167) makes body 125 at (3.3904, 108.091, 2.1167) makes body 126 at (3.3904, 128.091, 2.1167) in component "b front component"
combine "b front lines final combine feature" operation cut target body 102 tool bodies 103 104 105 106 107 108 109 110 111 112 113 114 115 116 117 118 119 120 121 122 123 124 125 126 in component "b front component"
sketch " back content" plane through (0, 0, 0) normal (0, 0, 1) x (1, 0, 0) in component "b back component"
  line L0 (182.01, 87.01) -> (182.01, 137.01) construction
  line L1 (182.01, 137.01) -> (92.01, 137.01) construction
  circle A0 centre (110.81, 112.01) radius 4
  line L2 (92.01, 137.01) -> (92.01, 87.01) construction
  line L3 (169.3373, 123.3571) -> (135.0459, 123.3571) construction
  line L4 (135.0459, 123.3571) -> (135.0459, 117.5676) construction
  line L5 (135.0459, 117.5676) -> (169.3373, 117.5676) construction
  line L6 (169.3373, 117.5676) -> (169.3373, 123.3571) construction
  line L7 (92.01, 87.01) -> (182.01, 87.01) construction
  point P0 (184.02, 85)
  dimension "d1816" = 5
  dimension "d502" = 90
  dimension "d503" = 50
  dimension "d696" = 25
  dimension "d1179" = 18.8
  dimension "d1562" = 8
  measures "d502" distance of L1.end L0.end
  measures "d503" distance of L0.start L0.end
  measures "d696" distance of A0.centre L1
  measures "d1179" distance of A0.centre L2
  measures "d1562" diameter of A0
sketch "b back lines" plane through (0, 0, 0) normal (0, 0, 1) x (1, 0, 0) in component "b back component"
  line L0 (95.185, 90.185) -> (101.91, 90.185)
  line L1 (101.91, 90.185) -> (101.91, 87.01)
  line L2 (101.91, 87.01) -> (112.11, 87.01)
  line L3 (112.11, 87.01) -> (112.11, 90.185)
  line L4 (112.11, 90.185) -> (121.91, 90.185)
  line L5 (121.91, 90.185) -> (121.91, 87.01)
  line L6 (121.91, 87.01) -> (132.11, 87.01)
  line L7 (132.11, 87.01) -> (132.11, 90.185)
  line L8 (132.11, 90.185) -> (141.91, 90.185)
  line L9 (141.91, 90.185) -> (141.91, 87.01)
  line L10 (141.91, 87.01) -> (152.11, 87.01)
  line L11 (152.11, 87.01) -> (152.11, 90.185)
  line L12 (152.11, 90.185) -> (161.91, 90.185)
  line L13 (161.91, 90.185) -> (161.91, 87.01)
  line L14 (161.91, 87.01) -> (172.11, 87.01)
  line L15 (172.11, 87.01) -> (172.11, 90.185)
  line L16 (172.11, 90.185) -> (178.835, 90.185)
  line L17 (178.835, 90.185) -> (178.835, 96.91)
  line L18 (178.835, 96.91) -> (182.01, 96.91)
  line L19 (182.01, 96.91) -> (182.01, 107.11)
  line L20 (182.01, 107.11) -> (178.835, 107.11)
  line L21 (178.835, 107.11) -> (178.835, 116.91)
  line L22 (178.835, 116.91) -> (182.01, 116.91)
  line L23 (182.01, 116.91) -> (182.01, 127.11)
  line L24 (182.01, 127.11) -> (178.835, 127.11)
  line L25 (178.835, 127.11) -> (178.835, 133.835)
  line L26 (95.185, 133.835) -> (101.91, 133.835)
  line L27 (101.91, 133.835) -> (101.91, 137.01)
  line L28 (101.91, 137.01) -> (112.11, 137.01)
  line L29 (112.11, 137.01) -> (112.11, 133.835)
  line L30 (112.11, 133.835) -> (121.91, 133.835)
  line L31 (121.91, 133.835) -> (121.91, 137.01)
  line L32 (121.91, 137.01) -> (132.11, 137.01)
  line L33 (132.11, 137.01) -> (132.11, 133.835)
  line L34 (132.11, 133.835) -> (141.91, 133.835)
  line L35 (141.91, 133.835) -> (141.91, 137.01)
  line L36 (141.91, 137.01) -> (152.11, 137.01)
  line L37 (152.11, 137.01) -> (152.11, 133.835)
  line L38 (152.11, 133.835) -> (161.91, 133.835)
  line L39 (161.91, 133.835) -> (161.91, 137.01)
  line L40 (161.91, 137.01) -> (172.11, 137.01)
  line L41 (172.11, 137.01) -> (172.11, 133.835)
  line L42 (172.11, 133.835) -> (178.835, 133.835)
  line L43 (95.185, 90.185) -> (95.185, 96.91)
  line L44 (95.185, 96.91) -> (92.01, 96.91)
  line L45 (92.01, 96.91) -> (92.01, 107.11)
  line L46 (92.01, 107.11) -> (95.185, 107.11)
  line L47 (95.185, 107.11) -> (95.185, 116.91)
  line L48 (95.185, 116.91) -> (92.01, 116.91)
  line L49 (92.01, 116.91) -> (92.01, 127.11)
  line L50 (92.01, 127.11) -> (95.185, 127.11)
  line L51 (95.185, 127.11) -> (95.185, 133.835)
sketch "b back circles" plane through (0, 0, 0) normal (0, 0, 1) x (1, 0, 0) in component "b back component"
  circle A0 centre (101.3194, 89.4744) radius 1.005
  circle A1 centre (112.7006, 89.4744) radius 1.005
  circle A2 centre (121.3194, 89.4744) radius 1.005
  circle A3 centre (132.7006, 89.4744) radius 1.005
  circle A4 centre (141.3194, 89.4744) radius 1.005
  circle A5 centre (152.7006, 89.4744) radius 1.005
  circle A6 centre (161.3194, 89.4744) radius 1.005
  circle A7 centre (172.7006, 89.4744) radius 1.005
  circle A8 centre (179.5456, 96.3194) radius 1.005
  circle A9 centre (179.5456, 107.7006) radius 1.005
  circle A10 centre (179.5456, 116.3194) radius 1.005
  circle A11 centre (179.5456, 127.7006) radius 1.005
  circle A12 centre (101.3194, 134.5456) radius 1.005
  circle A13 centre (112.7006, 134.5456) radius 1.005
  circle A14 centre (121.3194, 134.5456) radius 1.005
  circle A15 centre (132.7006, 134.5456) radius 1.005
  circle A16 centre (141.3194, 134.5456) radius 1.005
  circle A17 centre (152.7006, 134.5456) radius 1.005
  circle A18 centre (161.3194, 134.5456) radius 1.005
  circle A19 centre (172.7006, 134.5456) radius 1.005
  circle A20 centre (94.4744, 96.3194) radius 1.005
  circle A21 centre (94.4744, 107.7006) radius 1.005
  circle A22 centre (94.4744, 116.3194) radius 1.005
  circle A23 centre (94.4744, 127.7006) radius 1.005
extrude "b back lines lines extrude Feature" add sketch "b back lines" along normal blind 3.175 separate body makes body 127 in component "b back component"
extrude "b back circles circles extrude Feature" add sketch "b back circles" along normal blind 3.175 separate body makes body 128 at (93.53, 116.6631, 2.1167) makes body 129 at (93.53, 96.6631, 2.1167) makes body 130 at (161.7327, 135.4617, 2.1167) makes body 131 at (141.7327, 135.4617, 2.1167) makes body 132 at (122.0892, 135.1916, 2.1167) makes body 133 at (102.0892, 135.1916, 2.1167) makes body 134 at (179.959, 128.6167, 2.1167) makes body 135 at (178.6013, 108.0444, 2.1167) makes body 136 at (171.7563, 89.8181, 2.1167) makes body 137 at (151.7563, 89.8181, 2.1167) makes body 138 at (131.7563, 89.8181, 2.1167) makes body 139 at (111.7563, 89.8181, 2.1167) makes body 140 at (120.375, 89.8181, 2.1167) makes body 141 at (140.375, 89.8181, 2.1167) makes body 142 at (160.375, 89.8181, 2.1167) makes body 143 at (178.6013, 96.6631, 2.1167) makes body 144 at (178.6013, 116.6631, 2.1167) makes body 145 at (100.375, 89.8181, 2.1167) makes body 146 at (113.4705, 135.1916, 2.1167) makes body 147 at (133.114, 135.4617, 2.1167) makes body 148 at (153.114, 135.4617, 2.1167) makes body 149 at (173.114, 135.4617, 2.1167) makes body 150 at (93.53, 108.0444, 2.1167) makes body 151 at (93.53, 128.0444, 2.1167) in component "b back component"
combine "b back lines final combine feature" operation cut target body 127 tool bodies 128 129 130 131 132 133 134 135 136 137 138 139 140 141 142 143 144 145 146 147 148 149 150 151 in component "b back component"
component "b top component" placed x (1, 0, 0) y (0, 1, 0) z (0, 0, 1) at (0, 0, 0)
component "b bottom component" placed x (1, 0, 0) y (0, 1, 0) z (0, 0, 1) at (0, 0, 0)
component "b left component" placed x (1, 0, 0) y (0, 1, 0) z (0, 0, 1) at (0, 0, 0)
component "b right component" placed x (1, 0, 0) y (0, 1, 0) z (0, 0, 1) at (0, 0, 0)
component "b front component" placed x (1, 0, 0) y (0, 1, 0) z (0, 0, 1) at (0, 0, 0)
component "b back component" placed x (1, 0, 0) y (0, 1, 0) z (0, 0, 1) at (0, 0, 0)
equation "d1163 = length"
equation "d1817 = depth"
equation "d289 = platformGrommetMountDiameter"
equation "d422 = length"
equation "d423 = depth"
equation "d843 = toolDiameter"
equation "d1634 = pcbMountHoles"
equation "d1797 = ( depth - 26 mm ) / 2"
equation "d1798 = ( length - 58 mm ) / 2"
equation "d492 = length"
equation "d493 = height"
equation "d502 = length"
equation "d503 = height"
equation "d230 = length"
equation "d231 = height"
equation "d1827 = depth"
equation "d1829 = ventDiameter"
equation "d910 = depth"
equation "d911 = height"
equation "d1819 = ventDiameter"
equation "d467 = length"
equation "d468 = depth"
equation "d471 = ( depth - 26 mm ) / 2"
equation "d472 = ( length - 58 mm ) / 2"
equation "d479 = ventDiameter"